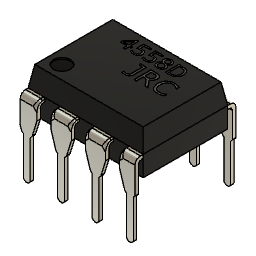
JRC_4558D (Autodesk Fusion 360 design; units mm, degrees)
Autodesk Fusion 360 part; units mm, degrees
note: some values were not read from the file. Chosen so that the rebuilt part matches the saved one: which bodies a step acts on; which pieces of a blend or face edit are solid.
sketch "Sketch1" plane through (0, 0, 0) normal (0, 0, 1) x (1, 0, 0)
  line L0 (4.25, -3.125) -> (-4.25, -3.125)
  line L1 (-4.25, -3.125) -> (-4.25, 3.125)
  line L2 (-4.25, 3.125) -> (4.25, 3.125)
  line L3 (4.25, 3.125) -> (4.25, -3.125)
  line L4 (4.25, -3.125) -> (-4.25, 3.125) construction
  line L5 (-4.25, -3.125) -> (4.25, 3.125) construction
  dimension "d1" = 8.5
  dimension "d2" = 6.25
  constraint horizontal L0
  constraint perpendicular L0 L1
  constraint parallel L0 L2
  constraint parallel L1 L3
  constraint coincident L4 origin
  constraint coincident L5 origin
  measures "d1" distance of L1.end L2.end
  measures "d2" distance of L0.end L1.end
extrude "Extrude1" add sketch "Sketch1" along normal blind 3 makes body 1
chamfer "Chamfer1" distance 0.25 distance2 1.5 1 faces at (1.4167, -1.0417, 3) on bodies 1
sketch "Sketch2" plane through (0, 0, 3) normal (0, 0, 1) x (-1, 0, 0)
  line L0 (4, 2.875) -> (-4, 2.875)
  line L1 (-4, 2.875) -> (-4, -2.875)
  line L2 (-4, -2.875) -> (4, -2.875)
  line L3 (4, -2.875) -> (4, 2.875)
  circle A0 centre (3, 1.875) radius 0.625
  line L4 (2.8903, -1.4982) -> (-2.8005, -1.4982) construction
  line L5 (-2.8005, -1.4982) -> (-2.8005, -2.3748) construction
  line L6 (-2.8005, -2.3748) -> (2.8903, -2.3748) construction
  line L7 (2.8903, -2.3748) -> (2.8903, -1.4982) construction
  line L8 (2.8903, 0.0018) -> (-2.8005, 0.0018) construction
  line L9 (-2.8005, 0.0018) -> (-2.8005, -0.8748) construction
  line L10 (-2.8005, -0.8748) -> (2.8903, -0.8748) construction
  line L11 (2.8903, -0.8748) -> (2.8903, 0.0018) construction
  dimension "d7" = 1.25
  dimension "d8" = 1
  dimension "d9" = 1
  dimension "d10" = 1
  dimension "d11" = 1.25
  text T0 "4558D" font "Verdana" height 1 align centre middle in box 5.6907 x 0.8765 at (2.8903, -1.4982) x (-1, 0) y (0, -1) spacing 1
  text T1 "JRC" font "Verdana" height 1.25 align right middle in box 5.6907 x 0.8765 at (2.8903, 0.0018) x (-1, 0) y (0, -1) spacing 1
  measures "d7" diameter of A0
  measures "d8" distance of L3 A0.centre
  measures "d9" distance of L0 A0.centre
extrude "Extrude2" add sketch "Sketch2" along normal blind 0.005 text T1 T0 bodies 1
sketch "Sketch3" plane through (0, 0, 0) normal (0, 0, -1) x (1, 0, 0)
  line L0 (-4.25, -3.125) -> (4.25, -3.125)
  line L1 (4.25, -3.125) -> (4.25, 3.125)
  line L2 (4.25, 3.125) -> (-4.25, 3.125)
  line L3 (-4.25, 3.125) -> (-4.25, -3.125)
  circle A0 centre (0, 0) radius 1.375
  dimension "d14" = 2.75
  constraint coincident A0.centre origin
  measures "d14" diameter of A0
extrude "Extrude3" cut sketch "Sketch3" against normal blind 0.1 contours A0 bodies 1
extrude "Extrude4" cut sketch "Sketch2" against normal blind 0.1 contours A0 bodies 1
sketch "Sketch4" plane through (0, -3.125, 0) normal (0, -1, 0) x (1, 0, 0)
  line L0 (4.25, 1.5) -> (-4.25, 1.5)
  line L1 (-4.25, 1.5) -> (-4.25, 0)
  line L2 (-4.25, 0) -> (4.25, 0)
  line L3 (4.25, 0) -> (4.25, 1.5)
  line L4 (-5, 1.5) -> (-3.5, 1.5)
  line L5 (-3.5, 1.5) -> (-3.5, 1.25)
  line L6 (-3.5, 1.25) -> (-5, 1.25)
  line L7 (-5, 1.25) -> (-5, 1.5)
  point P0 (-4.25, 1.375)
  dimension "d19" = 1.5
  dimension "d20" = 0.25
  constraint horizontal L4
  constraint vertical L5
  constraint horizontal L6
  constraint vertical L7
  constraint coincident L0 L4.start
  constraint coincident L1 P0
  measures "d19" distance of L4.start L4.end
  measures "d20" distance of L4.start L6.end
extrude "Extrude5" add sketch "Sketch4" along normal blind 0.6 separate body contours L0 L1 L4 L5 L6 | L1 L4 L6 L7 makes body 2
sketch "Sketch5" plane through (0, 0, 1.25) normal (0, 0, -1) x (1, 0, 0)
  line L0 (-5, 3.125) -> (-3.5, 3.125)
  line L1 (-3.5, 3.125) -> (-3.5, 3.725)
  line L2 (-3.5, 3.725) -> (-5, 3.725)
  line L3 (-5, 3.725) -> (-5, 3.125)
  line L4 (-5, 3.725) -> (-3.5, 3.725)
  line L5 (-3.5, 3.725) -> (-3.5, 3.475)
  line L6 (-3.5, 3.475) -> (-5, 3.475)
  line L7 (-5, 3.475) -> (-5, 3.725)
  dimension "d23" = 1.5
  dimension "d24" = 0.25
  constraint horizontal L4
  constraint vertical L5
  constraint horizontal L6
  constraint vertical L7
  constraint coincident L2.end L3.start
  measures "d23" distance of L2.end L1.end
  measures "d24" distance of L2.end L6.end
extrude "Extrude6" add sketch "Sketch5" along normal blind 5.25 contours L1 L2 L3 L4 L5 L6 L7 bodies 2
sketch "Sketch6" plane through (-5, 0, 0) normal (-1, 0, 0) x (0, -1, 0)
  line L0 (3.125, 1.5) -> (3.125, 1.25)
  line L1 (3.125, 1.25) -> (3.475, 1.25)
  line L2 (3.475, 1.25) -> (3.475, -4)
  line L3 (3.475, -4) -> (3.725, -4)
  line L4 (3.725, -4) -> (3.725, 1.5)
  line L5 (3.725, 1.5) -> (3.125, 1.5)
  line L6 (3.725, -4) -> (3.475, -4)
  line L7 (3.475, -4) -> (3.475, -1)
  line L8 (3.475, -1) -> (3.725, -1)
  line L9 (3.725, -1) -> (3.725, -4)
  dimension "d27" = 3
  constraint horizontal L6
  constraint vertical L7
  constraint horizontal L8
  constraint vertical L9
  constraint coincident L2 L7.end
  constraint coincident L3.end L4.start
  measures "d27" distance of L3.end L8.end
extrude "Extrude7" cut sketch "Sketch6" against normal blind 0.5 contours L2 L3 L4 L6 L7 L8 L9 bodies 2
chamfer "Chamfer2" distance 1.3 distance2 0.4 1 edges at (-5, -3.6, -1) measured on face at (-5, -3.6417, 0.5833) on bodies 2
chamfer "Chamfer3" distance 0.1 angle 45 1 edges at (-5, -3.425, 1.5) on bodies 2
fillet "Fillet1" radius 0.35 1 edges at (-4.6, -3.6, -1) on bodies 2
ref_plane "WorkPlane1" through (-4.25, -3.425, 0.85) normal (-1, 0, 0) x (0, 0, -1)
mirror "Mirror1" about plane through (-4.25, -3.425, 0.85) normal (-1, 0, 0) of "Extrude7"
chamfer "Chamfer4" distance 1.3 distance2 0.4 1 edges at (-3.5, -3.6, -1) measured on face at (-3.5, -3.6417, 0.5833) on bodies 2
fillet "Fillet2" radius 0.35 1 edges at (-3.9, -3.6, -1) on bodies 2
chamfer "Chamfer5" distance 0.1 distance2 0.1 1 edges at (-3.5, -3.425, 1.5) measured on face at (-3.5, -3.6417, 1.0167) on bodies 2
chamfer "Chamfer6" distance 0.15 angle 45 2 edges at (-4.5, -3.6, -4) (-4, -3.6, -4) on bodies 2
fillet "Fillet3" radius 0.4 3 edges at (-4.25, -3.725, 1.5) (-4.95, -3.725, 1.45) (-3.55, -3.725, 1.45) on bodies 2
fillet "Fillet4" radius 0.25 1 edges at (-4.25, -3.475, 1.25) on bodies 2
pattern_linear "R-Pattern1" count 4 spacing 2.54 along (1, 0, 0) of bodies 2 makes body 3 at (-1.5727, -3.725, -0.0661) makes body 4 at (0.9673, -3.725, -0.0661) makes body 5 at (3.5073, -3.725, -0.0661)
move_body "Move1" bodies 5 4 3 2 to x (1, 0, 0) y (0, 1, 0) z (0, 0, 1) at (0.5, 0, 0)
sketch "Sketch7" plane through (4.62, 0, 0) normal (1, 0, 0) x (0, 1, 0)
  ellipse E0 centre (-3.325, 0.8343) end of major axis (-3.325, 1.4) minor radius 0.4 (-3.325, 1.4) -> (-3.725, 0.8343) ccw
  line L0 (-3.725, 0.8343) -> (-3.725, 0.3)
  line L1 (-3.725, 0.3) -> (-3.475, 0.3)
  line L2 (-3.475, 0.3) -> (-3.475, 1)
  arc A0 (-3.225, 1.25) -> (-3.475, 1) centre (-3.225, 1) ccw
  line L3 (-3.225, 1.25) -> (-3.125, 1.25)
  line L4 (-3.125, 1.25) -> (-3.125, 1.4)
  line L5 (-3.125, 1.4) -> (-3.325, 1.4)
ref_plane "WorkPlane2" through (5.02, -3.425, 0.85) normal (1, 0, 0) x (0, 1, 0)
sketch "Sketch8" plane through (5.02, -3.425, 0.85) normal (1, 0, 0) x (0, 1, 0)
  line L0 (-1.9, 1.8) -> (0.9, 1.8)
  line L1 (0.9, 1.8) -> (0.9, -4.8)
  line L2 (0.9, -4.8) -> (-1.9, -4.8)
  line L3 (-1.9, -4.8) -> (-1.9, 1.8)
  constraint horizontal L0
  constraint vertical L1
  constraint horizontal L2
  constraint vertical L3
extrude "Extrude8" cut sketch "Sketch8" against normal blind 0.77 bodies 5
ref_plane "WorkPlane3" through (-5, -3.425, 0.85) normal (-1, 0, 0) x (0, 0, -1)
sketch "Sketch9" plane through (-5, -3.425, 0.85) normal (-1, 0, 0) x (0, -1, 0)
  line L0 (2.4479, 1.8592) -> (-1.6268, 1.8592)
  line L1 (-1.6268, 1.8592) -> (-1.6268, -5.2522)
  line L2 (-1.6268, -5.2522) -> (2.4479, -5.2522)
  line L3 (2.4479, -5.2522) -> (2.4479, 1.8592)
  constraint horizontal L0
  constraint vertical L1
  constraint horizontal L2
  constraint vertical L3
extrude "Extrude9" cut sketch "Sketch9" against normal blind 0.76 bodies 1 2
mirror "Mirror2" about plane through (0, 0, 0) normal (0, 1, 0) of bodies 2 5 3 4 makes body 6 at (-3.8267, 3.725, 0.2831) makes body 7 at (-1.0727, 3.725, -0.0661) makes body 8 at (1.4673, 3.725, -0.0661) makes body 9 at (3.8733, 3.725, 0.1762)
